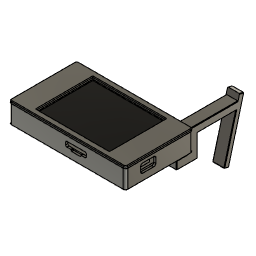
Cheap Yellow Display v16 (Autodesk Fusion 360 design; units mm, degrees)
part number: CYD
Autodesk Fusion 360 part; units mm, degrees
(part 1 of 2)
sketch "Sketch1" plane through (0, 0, 0) normal (0, 0, 1) x (1, 0, 0) in component "Display"
  line L0 (-39, 21) -> (39, 21) construction
  line L1 (39, 21) -> (39, -21) construction
  line L2 (39, -21) -> (-39, -21) construction
  line L3 (-39, -21) -> (-39, 21) construction
  line L4 (39, -25) -> (-39, -25)
  line L5 (-43, -21) -> (-43, 21)
  line L6 (-39, 25) -> (39, 25)
  line L7 (43, 21) -> (43, -21)
  arc A0 (43, 21) -> (39, 25) centre (39, 21) ccw
  arc A1 (39, -25) -> (43, -21) centre (39, -21) ccw
  arc A2 (-43, -21) -> (-39, -25) centre (-39, -21) ccw
  arc A3 (-39, 25) -> (-43, 21) centre (-39, 21) ccw
  circle A4 centre (-39, -21) radius 1.6
  circle A5 centre (39, -21) radius 1.6
  circle A6 centre (39, 21) radius 1.6
  circle A7 centre (-39, 21) radius 1.6
  dimension "d1" = 78
  dimension "d2" = 42
  dimension "d4" = 4
  dimension "d5" = 4
  dimension "d6" = 4
  dimension "d7" = 4
  dimension "d8" = 3.2
  dimension "d9" = 3.2
  dimension "d10" = 3.2
  dimension "d11" = 3.2
  constraint horizontal L0
  constraint vertical L1
  constraint horizontal L2
  constraint vertical L3
  constraint tangent L6 A0
  constraint tangent L7 A0
  constraint tangent L7 A1
  constraint tangent L4 A1
  constraint tangent L4 A2
  constraint tangent L5 A2
  constraint tangent L5 A3
  constraint tangent L6 A3
  constraint concentric A2 A4
  constraint concentric A1 A5
  constraint concentric A0 A6
  constraint concentric A3 A7
  measures "d1" distance of L0.start L0.end
  measures "d2" distance of L0.start L2.end
  measures "d4" radius of A0
  measures "d5" radius of A1
  measures "d6" radius of A2
  measures "d7" radius of A3
  measures "d8" diameter of A4
  measures "d9" diameter of A5
  measures "d10" diameter of A6
  measures "d11" diameter of A7
extrude "Extrude1" add sketch "Sketch1" along normal blind 1.5 makes body 1 in component "Display"
sketch "Sketch2" plane through (0, 0, 1.5) normal (0, 0, 1) x (-1, 0, 0) in component "Display"
  circle A0 centre (-39, 21) radius 1.6
  circle A1 centre (39, -21) radius 1.6
  circle A2 centre (39, 21) radius 1.6
  circle A3 centre (-39, -21) radius 1.6
  arc A4 (-43, -21) -> (-39, -25) centre (-39, -21) ccw
  line L0 (-39, -25) -> (39, -25)
  arc A5 (39, -25) -> (43, -21) centre (39, -21) ccw
  line L1 (43, -21) -> (43, 21)
  arc A6 (43, 21) -> (39, 25) centre (39, 21) ccw
  line L2 (39, 25) -> (-39, 25)
  arc A7 (-39, 25) -> (-43, 21) centre (-39, 21) ccw
  line L3 (-43, 21) -> (-43, -21)
  line L4 (34.5, -25) -> (-34.5, -25)
  line L5 (-34.5, -25) -> (-34.5, 25)
  line L6 (-34.5, 25) -> (34.5, 25)
  line L7 (34.5, 25) -> (34.5, -25)
  line L8 (41, 11) -> (38, 11)
  line L9 (38, 11) -> (38, 17)
  line L10 (38, 17) -> (41, 17)
  line L11 (41, 17) -> (41, 11)
  dimension "d14" = 69
  dimension "d15" = 50
  dimension "d16" = 8.5
  dimension "d19" = 6
  dimension "d20" = 2
  dimension "d21" = 8
  constraint horizontal L4
  constraint vertical L5
  constraint horizontal L6
  constraint vertical L7
  constraint horizontal L8
  constraint vertical L9
  constraint horizontal L10
  constraint vertical L11
  measures "d14" distance of L4.start L4.end
  measures "d15" distance of L4.start L6.end
  measures "d16" distance of L3 L5
  measures "d19" distance of L8.start L10.end
  measures "d20" distance of L1 L11
  measures "d21" distance of L2 L10
extrude "Extrude2" add sketch "Sketch2" along normal blind 3.5 contours L0 L2 L4 L5 L6 L7 bodies 1 in component "Display"
extrude "Extrude3" add sketch "Sketch2" along normal blind 0.5 contours L8 L9 L10 L11 bodies 1 in component "Display"
sketch "Sketch3" plane through (0, 0, 0) normal (0, 0, -1) x (1, 0, 0) in component "Display"
  circle A0 centre (39, 21) radius 1.6
  circle A1 centre (-39, -21) radius 1.6
  circle A2 centre (-39, 21) radius 1.6
  circle A3 centre (39, -21) radius 1.6
  arc A4 (39, -25) -> (43, -21) centre (39, -21) ccw
  line L0 (43, -21) -> (43, 21)
  arc A5 (43, 21) -> (39, 25) centre (39, 21) ccw
  line L1 (39, 25) -> (-39, 25)
  arc A6 (-39, 25) -> (-43, 21) centre (-39, 21) ccw
  line L2 (-43, 21) -> (-43, -21)
  arc A7 (-43, -21) -> (-39, -25) centre (-39, -21) ccw
  line L3 (-39, -25) -> (39, -25)
  line L4 (-17.6, -9) -> (-43, -9)
  line L5 (-43, -9) -> (-43, 9)
  line L6 (-43, 9) -> (-17.6, 9)
  line L7 (-17.6, 9) -> (-17.6, -9)
  line L8 (-10, 11.5) -> (-15, 11.5)
  line L9 (-15, 11.5) -> (-15, 16.5)
  line L10 (-15, 16.5) -> (-10, 16.5)
  line L11 (-10, 16.5) -> (-10, 11.5)
  line L12 (-31.9, -23.2) -> (-35.4, -23.2)
  line L13 (-35.4, -23.2) -> (-35.4, -17.2)
  line L14 (-35.4, -17.2) -> (-31.9, -17.2)
  line L15 (-31.9, -17.2) -> (-31.9, -23.2)
  line L16 (-31.4, -23.2) -> (-31.4, -17.2)
  line L17 (-31.4, -17.2) -> (-27.9, -17.2)
  line L18 (-27.9, -17.2) -> (-27.9, -23.2)
  line L19 (-27.9, -23.2) -> (-31.4, -23.2)
  line L20 (19, -23.8) -> (11.4, -23.8)
  line L21 (11.4, -23.8) -> (11.4, -20.6)
  line L22 (11.4, -20.6) -> (19, -20.6)
  line L23 (19, -20.6) -> (19, -23.8)
  line L24 (-36, -9) -> (-36, 9)
  line L25 (42, -14) -> (37.5, -14)
  line L26 (37.5, -14) -> (37.5, -4)
  line L27 (37.5, -4) -> (42, -4)
  line L28 (42, -4) -> (42, -14)
  line L29 (43.6, 5.4) -> (38.1, 5.4)
  line L30 (38.1, 5.4) -> (38.1, 13.2)
  line L31 (38.1, 13.2) -> (43.6, 13.2)
  line L32 (43.6, 13.2) -> (43.6, 5.4)
  line L33 (-22.8, 20.6) -> (-32.8, 20.6)
  line L34 (-32.8, 20.6) -> (-32.8, 24.9)
  line L35 (-32.8, 24.9) -> (-22.8, 24.9)
  line L36 (-22.8, 24.9) -> (-22.8, 20.6)
  line L37 (-16.8, 20.6) -> (-16.8, 24.9)
  line L38 (-16.8, 24.9) -> (-6.8, 24.9)
  line L39 (-6.8, 24.9) -> (-6.8, 20.6)
  line L40 (-6.8, 20.6) -> (-16.8, 20.6)
  line L41 (-2.6, 24.9) -> (12.4, 24.9)
  line L42 (12.4, 24.9) -> (12.4, 9.9)
  line L43 (12.4, 9.9) -> (-2.6, 9.9)
  line L44 (-2.6, 9.9) -> (-2.6, 24.9)
  dimension "d24" = 25.4
  dimension "d25" = 18
  dimension "d26" = 16
  dimension "d27" = 5
  dimension "d28" = 8.5
  dimension "d29" = 28
  dimension "d33" = 3.5
  dimension "d34" = 6
  dimension "d35" = 7.6
  dimension "d36" = 1.8
  dimension "d37" = 3.5
  dimension "d38" = 6
  dimension "d39" = 7.6
  dimension "d40" = 3.2
  dimension "d41" = 1.2
  dimension "d42" = 24
  dimension "d43" = 7
  dimension "d44" = 4.5
  dimension "d45" = 10
  dimension "d46" = 1
  dimension "d47" = 11
  dimension "d48" = 5.5
  dimension "d49" = 7.8
  dimension "d50" = 0.6
  dimension "d51" = 11.8
  dimension "d52" = 10
  dimension "d53" = 4.3
  dimension "d54" = 10.2
  dimension "d55" = 10
  dimension "d56" = 4.3
  dimension "d92" = 0.1
  dimension "d93" = 40.4
  constraint horizontal L4
  constraint vertical L5
  constraint horizontal L6
  constraint vertical L7
  constraint horizontal L8
  constraint vertical L9
  constraint horizontal L10
  constraint vertical L11
  constraint horizontal L12
  constraint vertical L13
  constraint horizontal L14
  constraint vertical L15
  constraint horizontal L19
  constraint vertical L16
  constraint horizontal L17
  constraint vertical L18
  constraint horizontal L20
  constraint vertical L21
  constraint horizontal L22
  constraint vertical L23
  constraint coincident L4 L24.start
  constraint coincident L6 L24.end
  constraint perpendicular L6 L24
  constraint horizontal L25
  constraint vertical L26
  constraint horizontal L27
  constraint vertical L28
  constraint horizontal L29
  constraint vertical L30
  constraint horizontal L31
  constraint vertical L32
  constraint horizontal L33
  constraint vertical L34
  constraint horizontal L35
  constraint vertical L36
  constraint horizontal L40
  constraint vertical L37
  constraint horizontal L38
  constraint vertical L39
  constraint horizontal L41
  constraint vertical L42
  constraint horizontal L43
  constraint vertical L44
  measures "d24" distance of L4.start L4.end
  measures "d25" distance of L4.start L6.end
  measures "d26" distance of L1 L6
  measures "d27" distance of L8.start L8.end
  measures "d28" distance of L1 L9.end
  measures "d29" distance of L2 L9.end
  measures "d33" distance of L12.start L12.end
  measures "d34" distance of L12.start L14.end
  measures "d35" horizontal distance of L2.end L12.end
  measures "d36" vertical distance of A7.end L12.end
  measures "d37" distance of L16.start L18.end
  measures "d38" distance of L18.end L17.end
  measures "d39" distance of L20.start L20.end
  measures "d40" distance of L20.start L22.end
  measures "d41" distance of L3 L20.end
  measures "d42" distance of A4.end L23
  measures "d43" distance of L5 L24
  measures "d44" distance of L25.start L25.end
  measures "d45" distance of L25.start L27.end
  measures "d46" distance of L0 L28
  measures "d47" distance of L3 L25
  measures "d48" distance of L29.start L29.end
  measures "d49" distance of L29.start L31.end
  measures "d50" distance of L0 L32
  measures "d51" distance of L1 L31
  measures "d52" distance of L33.start L33.end
  measures "d53" distance of L33.start L35.end
  measures "d54" distance of A6.end L34
  measures "d55" distance of L39.end L37.start
  measures "d56" distance of L38.end L39.end
  measures "d92" distance of L1 L41
  measures "d93" distance of L2 L44
extrude "Extrude4" add sketch "Sketch3" along normal blind 3 contours L4 L6 L7 L24 bodies 1 in component "Display"
extrude "Extrude5" add sketch "Sketch3" along normal blind 1 contours L2 L4 L5 L6 L24 bodies 1 in component "Display"
extrude "Extrude6" add sketch "Sketch3" along normal blind 3.5 contours L25 L26 L27 L28 | L33 L34 L35 L36 | L37 L38 L39 L40 bodies 1 in component "Display"
extrude "Extrude7" add sketch "Sketch3" along normal blind 1.5 contours L8 L9 L10 L11 bodies 1 in component "Display"
extrude "Extrude8" add sketch "Sketch3" along normal blind 2.5 contours L0 L29 L30 L31 | L0 L29 L31 L32 bodies 1 in component "Display"
extrude "Extrude9" add sketch "Sketch3" along normal blind 1.8 contours L41 L42 L43 L44 bodies 1 in component "Display"
extrude "Extrude10" add sketch "Sketch3" along normal blind 4.6 contours L20 L21 L22 L23 bodies 1 in component "Display"
extrude "Extrude11" add sketch "Sketch3" along normal blind 3.7 contours L12 L13 L14 L15 | L16 L17 L18 L19 bodies 1 in component "Display"
sketch "Sketch4" plane through (0, 0, -3.7) normal (0, 0, -1) x (1, 0, 0) in component "Display"
  line L0 (-27.9, -23.2) -> (-27.9, -17.2)
  line L1 (-27.9, -17.2) -> (-31.4, -17.2)
  line L2 (-31.4, -17.2) -> (-31.4, -23.2)
  line L3 (-31.4, -23.2) -> (-27.9, -23.2)
  line L4 (-28.9, -21.7) -> (-30.4, -21.7)
  line L5 (-30.4, -21.7) -> (-30.4, -18.7)
  line L6 (-30.4, -18.7) -> (-28.9, -18.7)
  line L7 (-28.9, -18.7) -> (-28.9, -21.7)
  line L8 (-29.65, -23.2) -> (-29.65, -24) construction
  line L9 (-31.4, -20.2) -> (-32, -20.2) construction
  line L10 (-35.4, -17.2) -> (-31.9, -17.2)
  line L11 (-31.9, -17.2) -> (-31.9, -23.2)
  line L12 (-35.4, -23.2) -> (-35.4, -17.2)
  line L13 (-31.9, -23.2) -> (-35.4, -23.2)
  line L14 (-33.65, -23.2) -> (-33.65, -24) construction
  line L15 (-35.4, -20.2) -> (-36, -20.2) construction
  line L16 (-34.4, -18.7) -> (-32.9, -18.7)
  line L17 (-32.9, -18.7) -> (-32.9, -21.7)
  line L18 (-32.9, -21.7) -> (-34.4, -21.7)
  line L19 (-34.4, -21.7) -> (-34.4, -18.7)
  dimension "d73" = 1.5
  dimension "d74" = 3
  dimension "d75" = 1.5
  dimension "d76" = 3
  constraint horizontal L4
  constraint vertical L5
  constraint horizontal L6
  constraint vertical L7
  constraint midpoint L3 L8.start
  constraint perpendicular L3 L8
  constraint midpoint L2 L9.start
  constraint perpendicular L2 L9
  constraint symmetric L5 L7 L8
  constraint symmetric L4 L6 L9
  constraint midpoint L13 L14.start
  constraint perpendicular L13 L14
  constraint midpoint L12 L15.start
  constraint perpendicular L12 L15
  constraint horizontal L18
  constraint vertical L19
  constraint horizontal L16
  constraint vertical L17
  constraint symmetric L15 L16 L18
  constraint symmetric L14 L17 L19
  measures "d73" distance of L4.start L4.end
  measures "d74" distance of L4.start L6.end
  measures "d75" distance of L17.end L18.end
  measures "d76" distance of L17.end L16.end
extrude "Extrude12" add sketch "Sketch4" along normal blind 1 contours L4 L5 L6 L7 | L16 L17 L18 L19 bodies 1 in component "Display"
sketch "Sketch5" plane through (0, 0, -1.5) normal (0, 0, -1) x (1, 0, 0) in component "Display"
  line L0 (-10, 16.5) -> (-15, 16.5)
  line L1 (-15, 16.5) -> (-15, 11.5)
  line L2 (-15, 11.5) -> (-10, 11.5)
  line L3 (-10, 11.5) -> (-10, 16.5)
  line L4 (-15, 16.5) -> (-10, 16.5)
  line L5 (-10, 16.5) -> (-10, 11.5)
  line L6 (-15, 11.5) -> (-15, 16.5)
  line L7 (-10, 11.5) -> (-15, 11.5)
  line L8 (-15, 16.5) -> (-10, 11.5) construction
  circle A0 centre (-12.5, 14) radius 2
  dimension "d79" = 4
  constraint coincident L0.end L1.start
  constraint coincident L2.end L3.start
  constraint midpoint L8 A0.centre
  measures "d79" diameter of A0
extrude "Extrude13" add sketch "Sketch5" along normal blind 0.1 contours A0 bodies 1 in component "Display"
sketch "Sketch6" plane through (0, 0, 5) normal (0, 0, 1) x (-1, 0, 0) in component "Display"
  line L0 (34.5, 25) -> (-34.5, 25)
  line L1 (-34.5, 25) -> (-34.5, -25)
  line L2 (-34.5, -25) -> (34.5, -25)
  line L3 (34.5, -25) -> (34.5, 25)
  line L4 (32, -22.5) -> (-27, -22.5)
  line L5 (-27, -22.5) -> (-27, 22.5)
  line L6 (-27, 22.5) -> (32, 22.5)
  line L7 (32, 22.5) -> (32, -22.5)
  line L8 (34.5, 0) -> (42, 0) construction
  line L9 (43, -21) -> (43, 21)
  line L10 (43, -9.5) -> (36.8, -9.5)
  line L11 (36.8, -9.5) -> (36.8, 9.5)
  line L12 (36.8, 9.5) -> (43, 9.5)
  line L13 (43, 9.5) -> (43, -9.5)
  dimension "d82" = 59
  dimension "d83" = 45
  dimension "d84" = 2.5
  dimension "d85" = 6.2
  dimension "d86" = 19
  constraint horizontal L4
  constraint vertical L5
  constraint horizontal L6
  constraint vertical L7
  constraint midpoint L3 L8.start
  constraint perpendicular L3 L8
  constraint symmetric L4 L6 L8
  constraint horizontal L10
  constraint vertical L11
  constraint horizontal L12
  constraint vertical L13
  constraint coincident L9 L10.start
  constraint symmetric L8 L10 L12
  measures "d82" distance of L4.start L4.end
  measures "d83" distance of L4.start L6.end
  measures "d84" distance of L3 L7
  measures "d85" distance of L10.start L10.end
  measures "d86" distance of L10.start L12.end
extrude "Extrude14" add sketch "Sketch6" along normal blind 0.1 contours L4 L5 L6 L7 bodies 1 in component "Display"
extrude "Extrude15" cut sketch "Sketch6" against normal up to surface (1.5 mm away) from surface at -3.5 contours L9 L10 L11 L12 L13 bodies 1 in component "Display"
sketch "Sketch1 (2)" plane through (0, 0, 5) normal (0, 0, 1) x (-1, 0, 0) in component "case front"
  line L0 (32, 22.5) -> (32, -22.5)
  line L1 (32, -22.5) -> (-27, -22.5)
  line L2 (-27, -22.5) -> (-27, 22.5)
  line L3 (-27, 22.5) -> (32, 22.5)
  line L4 (34.5, 25) -> (-34.5, 25)
  line L5 (-34.5, 25) -> (-34.5, -25)
  line L6 (-34.5, -25) -> (34.5, -25)
  line L7 (34.5, -25) -> (34.5, 25)
  line L8 (-27, 22.5) -> (-27, -22.5)
  line L9 (-27, -22.5) -> (32, -22.5)
  line L10 (32, -22.5) -> (32, 22.5)
  line L11 (32, 22.5) -> (-27, 22.5)
  line L12 (-27, 22.5) -> (-27, -22.5)
  line L13 (-27, -22.5) -> (32, -22.5)
  line L14 (32, -22.5) -> (32, 22.5)
  line L15 (-28, 23.5) -> (33, 23.5)
  line L16 (33, 23.5) -> (33, -23.5)
  line L17 (33, -23.5) -> (-28, -23.5)
  line L18 (-28, -23.5) -> (-28, 23.5)
  line L19 (43, -21) -> (43, -9.5) construction
  line L20 (-34.5, -25) -> (34.5, -25)
  line L21 (34.5, 25) -> (-34.5, 25)
  line L22 (-43, 21) -> (-43, -21) construction
  line L23 (49.5, -28.5) -> (-44.5, -28.5)
  line L24 (-46.5, -26.5) -> (-46.5, 26.5)
  line L25 (-44.5, 28.5) -> (49.5, 28.5)
  line L26 (51.5, 26.5) -> (51.5, -26.5)
  arc A0 (51.5, 26.5) -> (49.5, 28.5) centre (49.5, 26.5) ccw
  arc A1 (49.5, -28.5) -> (51.5, -26.5) centre (49.5, -26.5) ccw
  arc A2 (-46.5, -26.5) -> (-44.5, -28.5) centre (-44.5, -26.5) ccw
  arc A3 (-44.5, 28.5) -> (-46.5, 26.5) centre (-44.5, 26.5) ccw
  dimension "d94" = -1
  dimension "d99" = 2
  dimension "d100" = 2
  dimension "d101" = 2
  dimension "d102" = 2
  dimension "d105" = 18.5
  dimension "d106" = 18.5
  dimension "BORDER_H" = 5
  dimension "d108" = 5
  constraint horizontal L23
  constraint vertical L24
  constraint horizontal L25
  constraint vertical L26
  constraint tangent L26 A0
  constraint tangent L25 A0
  constraint tangent L26 A1
  constraint tangent L23 A1
  constraint tangent L23 A2
  constraint tangent L24 A2
  constraint tangent L24 A3
  constraint tangent L25 A3
  measures "d99" radius of A0
  measures "d100" radius of A1
  measures "d101" radius of A2
  measures "d102" radius of A3
  measures "d105" distance of L16 L26
  measures "d106" distance of L18 L24
  measures "BORDER_H" distance of L17 L23
  measures "d108" distance of L15 L25
extrude "Extrude1'" add sketch "Sketch1 (2)" along normal blind 1.8 separate body contours L4 L5 L6 L7 L20 L21 | L23 L24 L25 L26 A0 A1 A2 A3 makes body 2 in component "case front"
sketch "Sketch2 (2)" plane through (0, 0, 5) normal (0, 0, -1) x (1, 0, 0) in component "case front"
  line L0 (28, -23.5) -> (-33, -23.5)
  line L1 (-33, -23.5) -> (-33, 23.5)
  line L2 (-33, 23.5) -> (28, 23.5)
  line L3 (28, 23.5) -> (28, -23.5)
  arc A0 (-49.5, 28.5) -> (-51.5, 26.5) centre (-49.5, 26.5) ccw
  line L4 (-51.5, 26.5) -> (-51.5, -26.5)
  arc A1 (-51.5, -26.5) -> (-49.5, -28.5) centre (-49.5, -26.5) ccw
  line L5 (-49.5, -28.5) -> (44.5, -28.5)
  arc A2 (44.5, -28.5) -> (46.5, -26.5) centre (44.5, -26.5) ccw
  line L6 (46.5, -26.5) -> (46.5, 26.5)
  arc A3 (46.5, 26.5) -> (44.5, 28.5) centre (44.5, 26.5) ccw
  line L7 (44.5, 28.5) -> (-49.5, 28.5)
  line L8 (44.5, 28.5) -> (-49.5, 28.5)
  arc A4 (46.5, 26.5) -> (44.5, 28.5) centre (44.5, 26.5) ccw
  line L9 (46.5, -26.5) -> (46.5, 26.5)
  arc A5 (44.5, -28.5) -> (46.5, -26.5) centre (44.5, -26.5) ccw
  line L10 (-49.5, -28.5) -> (44.5, -28.5)
  arc A6 (-51.5, -26.5) -> (-49.5, -28.5) centre (-49.5, -26.5) ccw
  line L11 (-51.5, 26.5) -> (-51.5, -26.5)
  arc A7 (-49.5, 28.5) -> (-51.5, 26.5) centre (-49.5, 26.5) ccw
  line L12 (-50.5, 26.5) -> (-50.5, -26.5)
  arc A8 (-50.5, -26.5) -> (-49.5, -27.5) centre (-49.5, -26.5) ccw
  line L13 (-49.5, -27.5) -> (44.5, -27.5)
  arc A9 (44.5, -27.5) -> (45.5, -26.5) centre (44.5, -26.5) ccw
  line L14 (45.5, -26.5) -> (45.5, 26.5)
  arc A10 (45.5, 26.5) -> (44.5, 27.5) centre (44.5, 26.5) ccw
  line L15 (44.5, 27.5) -> (-49.5, 27.5)
  arc A11 (-49.5, 27.5) -> (-50.5, 26.5) centre (-49.5, 26.5) ccw
  line L16 (-49.7, 26.5) -> (-49.7, -26.5)
  arc A12 (-49.7, -26.5) -> (-49.5, -26.7) centre (-49.5, -26.5) ccw
  line L17 (-49.5, -26.7) -> (44.5, -26.7)
  arc A13 (44.5, -26.7) -> (44.7, -26.5) centre (44.5, -26.5) ccw
  line L18 (44.7, -26.5) -> (44.7, 26.5)
  arc A14 (44.7, 26.5) -> (44.5, 26.7) centre (44.5, 26.5) ccw
  line L19 (44.5, 26.7) -> (-49.5, 26.7)
  arc A15 (-49.5, 26.7) -> (-49.7, 26.5) centre (-49.5, 26.5) ccw
  circle A16 centre (-39, -21) radius 1.6
  circle A17 centre (-39, 21) radius 1.6
  circle A18 centre (39, 21) radius 1.6
  circle A19 centre (39, -21) radius 1.6
  circle A20 centre (39, 21) radius 3.6
  circle A21 centre (-39, 21) radius 3.6
  circle A22 centre (-39, -21) radius 3.6
  circle A23 centre (39, -21) radius 3.6
  circle A24 centre (-39, 21) radius 1.4
  circle A25 centre (39, 21) radius 1.4
  circle A26 centre (39, -21) radius 1.4
  circle A27 centre (-39, -21) radius 1.4
  dimension "d110" = -1
  dimension "d112" = 2
  dimension "d113" = 2
  dimension "d114" = 2
  dimension "d115" = 2
  dimension "d116" = -0.2
  dimension "d117" = -0.2
  dimension "d118" = -0.2
  dimension "d119" = -0.2
extrude "Extrude2'" add sketch "Sketch2 (2)" along normal blind 1 contours L12 A8 L13 A9 L14 A10 L15 A11 bodies 2 in component "case front"
extrude "Extrude3'" add sketch "Sketch2 (2)" along normal up to surface (5 mm away) contours A16 | A17 | A18 | A19 | A24 | A25 | A26 | A27 bodies 2 in component "case front"
extrude "Extrude4'" add sketch "Sketch2 (2)" along normal up to surface (3.5 mm away) contours A20 | A21 | A22 | A23 bodies 2 in component "case front"
chamfer "Chamfer1" distance 0.6 angle 45 12 edges at (45.9142, 27.9142, 6.8) (-2.5, 28.5, 6.8) (-50.9142, 27.9142, 6.8) (-51.5, 0, 6.8) (-50.9142, -27.9142, 6.8) (-2.5, -28.5, 6.8) (45.9142, -27.9142, 6.8) (46.5, 0, 6.8) (-33, 0, 6.8) (-2.5, -23.5, 6.8) (-2.5, 23.5, 6.8) (28, 0, 6.8) on bodies 2 in component "case front"
sketch "Sketch1 (3)" plane through (0, 0, 4) normal (0, 0, -1) x (1, 0, 0) in component "case rear"
  arc A0 (-49.5, 26.7) -> (-49.7, 26.5) centre (-49.5, 26.5) ccw
  line L0 (-49.5, 26.7) -> (44.5, 26.7)
  arc A1 (44.7, 26.5) -> (44.5, 26.7) centre (44.5, 26.5) ccw
  line L1 (44.7, 26.5) -> (44.7, -26.5)
  arc A2 (44.5, -26.7) -> (44.7, -26.5) centre (44.5, -26.5) ccw
  line L2 (44.5, -26.7) -> (-49.5, -26.7)
  arc A3 (-49.7, -26.5) -> (-49.5, -26.7) centre (-49.5, -26.5) ccw
  line L3 (-49.7, -26.5) -> (-49.7, 26.5)
  arc A4 (-49.5, 27.5) -> (-50.5, 26.5) centre (-49.5, 26.5) ccw
  line L4 (-50.5, 26.5) -> (-50.5, -26.5)
  arc A5 (-50.5, -26.5) -> (-49.5, -27.5) centre (-49.5, -26.5) ccw
  line L5 (-49.5, -27.5) -> (44.5, -27.5)
  arc A6 (44.5, -27.5) -> (45.5, -26.5) centre (44.5, -26.5) ccw
  line L6 (45.5, -26.5) -> (45.5, 26.5)
  arc A7 (45.5, 26.5) -> (44.5, 27.5) centre (44.5, 26.5) ccw
  line L7 (44.5, 27.5) -> (-49.5, 27.5)
  arc A8 (-51.5, -26.5) -> (-49.5, -28.5) centre (-49.5, -26.5) ccw
  line L8 (-49.5, -28.5) -> (44.5, -28.5)
  line L9 (-51.5, 26.5) -> (-51.5, -26.5)
  arc A9 (44.5, -28.5) -> (46.5, -26.5) centre (44.5, -26.5) ccw
  line L10 (46.5, -26.5) -> (46.5, 26.5)
  arc A10 (46.5, 26.5) -> (44.5, 28.5) centre (44.5, 26.5) ccw
  line L11 (44.5, 28.5) -> (-49.5, 28.5)
  arc A11 (-49.5, 28.5) -> (-51.5, 26.5) centre (-49.5, 26.5) ccw
  line L12 (-49.7, -26.5) -> (-49.7, 26.5)
  arc A12 (-49.5, 26.7) -> (-49.7, 26.5) centre (-49.5, 26.5) ccw
  line L13 (-49.5, 26.7) -> (44.5, 26.7)
  arc A13 (44.7, 26.5) -> (44.5, 26.7) centre (44.5, 26.5) ccw
  line L14 (44.7, 26.5) -> (44.7, -26.5)
  arc A14 (44.5, -26.7) -> (44.7, -26.5) centre (44.5, -26.5) ccw
  line L15 (44.5, -26.7) -> (-49.5, -26.7)
  arc A15 (-49.7, -26.5) -> (-49.5, -26.7) centre (-49.5, -26.5) ccw
  arc A16 (44.5, -27.7) -> (45.7, -26.5) centre (44.5, -26.5) ccw
  line L16 (45.7, -26.5) -> (45.7, 26.5)
  arc A17 (45.7, 26.5) -> (44.5, 27.7) centre (44.5, 26.5) ccw
  line L17 (44.5, 27.7) -> (-49.5, 27.7)
  arc A18 (-49.5, 27.7) -> (-50.7, 26.5) centre (-49.5, 26.5) ccw
  line L18 (-50.7, 26.5) -> (-50.7, -26.5)
  arc A19 (-50.7, -26.5) -> (-49.5, -27.7) centre (-49.5, -26.5) ccw
  line L19 (-49.5, -27.7) -> (44.5, -27.7)
  dimension "d127" = -0.8
extrude "Extrude1''" add sketch "Sketch1 (3)" against normal up to surface (0.9 mm away) separate body contours A8 L8 L9 A9 L10 A10 L11 A11 makes body 3 in component "case rear"
extrude "Extrude2''" add sketch "Sketch1 (3)" along normal blind 15 contours A4 L4 A5 L5 A6 L6 A7 L7 | A8 L8 L9 A9 L10 A10 L11 A11 | A16 L16 A17 L17 A18 L18 A19 L19 bodies 3 in component "case rear"
sketch "Sketch2 (3)" plane through (0, 0, -11) normal (0, 0, -1) x (1, 0, 0) in component "case rear"
  arc A0 (-49.5, 26.7) -> (-49.7, 26.5) centre (-49.5, 26.5) ccw
  line L0 (-49.5, 26.7) -> (44.5, 26.7)
  arc A1 (44.7, 26.5) -> (44.5, 26.7) centre (44.5, 26.5) ccw
  line L1 (44.7, 26.5) -> (44.7, -26.5)
  arc A2 (44.5, -26.7) -> (44.7, -26.5) centre (44.5, -26.5) ccw
  line L2 (44.5, -26.7) -> (-49.5, -26.7)
  arc A3 (-49.7, -26.5) -> (-49.5, -26.7) centre (-49.5, -26.5) ccw
  line L3 (-49.7, -26.5) -> (-49.7, 26.5)
  arc A4 (-49.5, 28.5) -> (-51.5, 26.5) centre (-49.5, 26.5) ccw
  line L4 (-51.5, 26.5) -> (-51.5, -26.5)
  arc A5 (-51.5, -26.5) -> (-49.5, -28.5) centre (-49.5, -26.5) ccw
  line L5 (-49.5, -28.5) -> (44.5, -28.5)
  arc A6 (44.5, -28.5) -> (46.5, -26.5) centre (44.5, -26.5) ccw
  line L6 (46.5, -26.5) -> (46.5, 26.5)
  arc A7 (46.5, 26.5) -> (44.5, 28.5) centre (44.5, 26.5) ccw
  line L7 (44.5, 28.5) -> (-49.5, 28.5)
  line L8 (46.5, -26.5) -> (46.5, 26.5)
  arc A8 (46.5, 26.5) -> (44.5, 28.5) centre (44.5, 26.5) ccw
  line L9 (44.5, 28.5) -> (-49.5, 28.5)
  arc A9 (-49.5, 28.5) -> (-51.5, 26.5) centre (-49.5, 26.5) ccw
  line L10 (-51.5, 26.5) -> (-51.5, -26.5)
  arc A10 (-51.5, -26.5) -> (-49.5, -28.5) centre (-49.5, -26.5) ccw
  arc A11 (44.5, -28.5) -> (46.5, -26.5) centre (44.5, -26.5) ccw
  line L11 (-49.5, -28.5) -> (44.5, -28.5)
  circle A12 centre (-39, -21) radius 1.6
  circle A13 centre (39, -21) radius 1.6
  circle A14 centre (39, 21) radius 1.6
  circle A15 centre (-39, 21) radius 1.6
  circle A16 centre (-44, -21) radius 3.4
  circle A17 centre (-44, 21) radius 3.4
  circle A18 centre (39, -21) radius 3.4
  circle A19 centre (39, 21) radius 3.4
  line L12 (-44, -21) -> (39, -21)
  line L13 (39, -21) -> (39, 21)
  line L14 (39, 21) -> (-44, 21)
  line L15 (-44, 21) -> (-44, -21)
  circle A20 centre (-44, -21) radius 5
  circle A21 centre (-44, 21) radius 5
  circle A22 centre (39, -21) radius 5
  circle A23 centre (39, 21) radius 5
  point P0 (39, -21)
  dimension "d132" = 1.8
  dimension "d133" = 1.8
  dimension "d134" = 1.8
  dimension "d135" = 1.8
  dimension "d210" = 10
  dimension "d211" = 10
  dimension "d212" = 10
  dimension "d213" = 10
  constraint horizontal L12
  constraint vertical L13
  constraint horizontal L14
  constraint vertical L15
  constraint coincident A14.centre A19.centre
  constraint coincident A16.centre L12.start
  constraint concentric A16 A20
  constraint concentric A17 A21
  constraint concentric A13 A22
  constraint coincident P0 A13.centre
  measures "d210" diameter of A20
  measures "d211" diameter of A21
  measures "d212" diameter of A22
  measures "d213" diameter of A23
extrude "Extrude3''" add sketch "Sketch2 (3)" against normal up to surface (10.9 mm away) separate body contours A16 L12 L15 | A16 L12 L15 | A13 A18 L12 L13 | A13 A18 L12 L13 | A13 L12 L13 | A13 L12 L13 | A17 L14 L15 | A17 L14 L15 | A14 A19 L13 L14 | A14 A19 L13 L14 | A14 L13 L14 | A14 L13 L14 makes body 4 at (-40.6169, 20.6615, -7.3667) makes body 5 at (42.3831, 20.6615, -7.3667) makes body 6 at (-40.6169, -21.3385, -7.3667) makes body 7 at (42.3831, -21.3385, -7.3667) in component "case rear"
extrude "Extrude4''" add sketch "Sketch2 (3)" against normal blind 1.8 contours A0 L0 A1 L1 A2 L2 A3 L3 | A12 L12 A20 | A12 L12 A20 | A12 A15 L12 L13 L14 L15 A20 A21 A22 A23 | A12 L12 A20 | A12 A16 L15 A20 | A12 A16 L15 A20 | A12 L12 A20 | A18 L12 L13 A22 | A18 L12 L13 A22 | A15 A17 L15 A21 | A15 A17 L15 A21 | A19 L13 L14 A23 | A19 L13 L14 A23 | A15 L14 A21 | A15 L14 A21 | A15 L14 A21 | A15 L14 A21 bodies 3 4 5 6 7 in component "case rear"
sketch "Sketch3 (2)" plane through (46.5, 0, 0) normal (1, 0, 0) x (0, 1, 0) in component "case rear"
  line L0 (26.5, 4.9) -> (-26.5, 4.9)
  line L1 (-26.5, 4.9) -> (-26.5, -11)
  line L2 (-26.5, -11) -> (26.5, -11)
  line L3 (26.5, -11) -> (26.5, 4.9)
  line L4 (-5.4, 0) -> (-13.2, 0)
  line L5 (-13.2, 0) -> (-13.2, -2.5)
  line L6 (-13.2, -2.5) -> (-5.4, -2.5)
  line L7 (-5.4, -2.5) -> (-5.4, 0)
  line L8 (-14.1, -5) -> (-4.5, -5)
  line L9 (-2.9, -3.4) -> (-2.9, 0.9)
  line L10 (-4.5, 2.5) -> (-14.1, 2.5)
  line L11 (-15.7, 0.9) -> (-15.7, -3.4)
  arc A0 (-14.1, 2.5) -> (-15.7, 0.9) centre (-14.1, 0.9) ccw
  arc A1 (-2.9, 0.9) -> (-4.5, 2.5) centre (-4.5, 0.9) ccw
  arc A2 (-4.5, -5) -> (-2.9, -3.4) centre (-4.5, -3.4) ccw
  arc A3 (-15.7, -3.4) -> (-14.1, -5) centre (-14.1, -3.4) ccw
  dimension "d141" = 1.6
  dimension "d142" = 1.6
  dimension "d143" = 1.6
  dimension "d144" = 1.6
  constraint tangent L11 A0
  constraint tangent L10 A0
  constraint tangent L10 A1
  constraint tangent L9 A1
  constraint tangent L9 A2
  constraint tangent L8 A2
  constraint tangent L8 A3
  constraint tangent L11 A3
  measures "d141" radius of A0
  measures "d142" radius of A1
  measures "d143" radius of A2
  measures "d144" radius of A3
extrude "Extrude5'" cut sketch "Sketch3 (2)" against normal up to surface (1.8 mm away) contours L4 L5 L6 L7 | L8 L9 L10 L11 A0 A1 A2 A3 bodies 3 in component "case rear"
chamfer "Chamfer1'" distance 0.6 angle 45 8 edges at (-2.5, 28.5, -11) (45.9142, 27.9142, -11) (46.5, 0, -11) (45.9142, -27.9142, -11) (-2.5, -28.5, -11) (-50.9142, -27.9142, -11) (-51.5, 0, -11) (-50.9142, 27.9142, -11) on bodies 3 in component "case rear"
ref_plane "WorkPlane1" through (-2.5, 0, 5.9) normal (1, 0, 0) x (0, 1, 0) in component "case front"
sketch "Sketch3 (3)" plane through (-2.5, 0, 5.6) normal (1, 0, 0) x (0, 1, 0) in component "case front"
  line L0 (27.5, -0.6) -> (27.5, -1.6)
  line L1 (-26.5, -0.6) -> (26.5, -0.6)
  line L2 (26.5971, -0.6) -> (25.0971, -0.6)
  line L3 (25.0971, -0.6) -> (25.5097, -3.8)
  line L4 (25.5097, -3.8) -> (26.5971, -3.8)
  line L5 (26.5971, -3.8) -> (26.5971, -0.6)
  line L6 (25.6, -3.0789) -> (26.7, -3.0789) construction
  line L7 (26.2971, -2.2066) -> (26.2971, -1.3) construction
  circle A0 centre (26.2971, -3.0789) radius 0.781
  line L8 (26.5, -0.6) -> (-26.5, -0.6)
  line L9 (0, -0.6) -> (0, 4.4) construction
  line L10 (-25.0971, -0.6) -> (-25.5097, -3.8)
  line L11 (-26.2971, -2.2066) -> (-26.1739, -0.589) construction
  line L12 (-25.5097, -3.8) -> (-26.5971, -3.8)
  line L13 (-26.5, -0.6) -> (-26.5, -1.6)
  line L14 (-26.5981, -0.6) -> (-25.0971, -0.6)
  line L15 (-25.6, -3.0789) -> (-26.7, -3.0789) construction
  circle A1 centre (-26.2971, -3.0789) radius 0.781
  line L16 (-26.5971, -3.8) -> (-26.5981, -0.6)
  line L17 (26.7, -0.6) -> (26.7, -1.6)
  point P0 (-26.5, -0.6)
  point P1 (-26.5, -0.6)
  dimension "d148" = 1.5
  dimension "d149" = 3.2
  dimension "d152" = 5
  constraint horizontal L2
  constraint horizontal L4
  constraint vertical L5
  constraint coincident L6 A0.centre
  constraint coincident L7 A0.centre
  constraint coincident L4.end A0
  constraint midpoint L8 L9.start
  constraint perpendicular L8 L9
  constraint coincident L3.end L4.start
  constraint symmetric L2.end L9 L10.start
  constraint symmetric L3.end L9 L10.end
  constraint symmetric L4.end L9 L12.end
  constraint symmetric L6.start L9 L15.start
  constraint symmetric L6.end L9 L15.end
  constraint symmetric L7.start L9 L11.start
  constraint symmetric A0 L9 A1
  constraint collinear L2 L8
  measures "d148" distance of L2.start L2.end
  measures "d149" distance of L2.start L4.end
  measures "d152" distance of L9.start L9.end
extrude "Extrude5''" add sketch "Sketch3 (3)" along normal mid plane 75 contours L1 L8 L10 L12 L14 A1 L16 | A1 L16 | L12 A1 L16 | L1 L2 L3 L4 L5 A0 L8 | L4 L5 A0 | L5 A0 bodies 2 in component "case front"
sketch "Sketch4 (2)" plane through (-2.5, 0, 5.6) normal (1, 0, 0) x (0, 1, 0) in component "case rear"
  line L0 (26.7, -1.6) -> (26.7, -14.8)
  line L1 (26.5971, -3.8) -> (25.5097, -3.8)
  line L2 (27.7, -1.6) -> (26.5, -1.6)
  line L3 (26.7, -1.6) -> (26.9, -1.6)
  line L4 (26.7, -1.6) -> (26.7, -2.15)
  line L5 (26.7, -2.15) -> (26.9, -1.6)
  line L6 (0, -0.6) -> (0, 4.4)
  line L7 (-26.7, -1.6) -> (-26.9, -1.6)
  line L8 (-26.7, -1.6) -> (-26.7, -2.15)
  line L9 (-26.7, -2.15) -> (-26.9, -1.6)
  line L10 (-26.7, -1.6) -> (-26.7, -14.8)
  circle A0 centre (26.2971, -3.0789) radius 0.781
  circle A1 centre (26.2971, -3.0789) radius 0.831
  circle A2 centre (-26.2971, -3.0789) radius 0.831
  line L11 (-26.7, -1.6) -> (-26.7, -14.8)
  point P0 (-26.5, -1.6)
  point P1 (26.5971, -2.3578)
  point P2 (26.5971, -0.6)
  dimension "d158" = 0.05
  constraint coincident L0.start L3.start
  constraint coincident L2 L3.end
  constraint perpendicular L0 L3
  constraint coincident L0 L4.end
  constraint symmetric L0.start L6 L7.start
  constraint symmetric L0.end L6 L10.end
  constraint symmetric L2.end L6 P0
  constraint symmetric L3.end L6 L7.end
  constraint symmetric L4.end L6 L8.end
  constraint symmetric L6 A1 A2
extrude "Extrude6'" cut sketch "Sketch4 (2)" along normal mid plane 76 contours L0 L2 L3 L4 L5 | L0 A0 A1 | L0 A0 | L7 L8 L9 L10 L11 | L10 A2 L11 picked at (-26.8255, -3.1751) bodies 3 in component "case rear"
fillet "Fillet1" radius 1.2 4 edges at (-42.3564, 19.6982, 5) (-42.3564, -22.3018, 5) (35.6436, -22.3018, 5) (35.6436, 19.6982, 5) on bodies 2 in component "case front"
sketch "Sketch5 (2)" plane through (0, -28.5, 0) normal (0, -1, 0) x (1, 0, 0) in component "case rear"
  line L0 (-49.5, -10.4) -> (44.5, -10.4)
  line L1 (44.5, -10.4) -> (44.5, 4.9)
  line L2 (44.5, 4.9) -> (-49.5, 4.9)
  line L3 (-49.5, 4.9) -> (-49.5, -10.4)
  line L4 (-2.6, 0) -> (-2.6, -1.8)
  line L5 (12.4, -1.8) -> (-2.6, -1.8)
  line L6 (12.4, 0) -> (-2.6, 0)
  line L7 (-2.6, 0) -> (-2.6, -1.8)
  line L8 (-2.6, -1.8) -> (12.4, -1.8)
  line L9 (12.4, -1.8) -> (12.4, 0)
  line L10 (-2.8, -3.4) -> (12.6, -3.4) construction
  line L11 (13.6, -2.4) -> (13.6, -0.2)
  line L12 (12.6, 0.8) -> (-2.8, 0.8)
  line L13 (-3.8, -0.2) -> (-3.8, -2.4)
  arc A0 (-2.8, 0.8) -> (-3.8, -0.2) centre (-2.8, -0.2) ccw
  arc A1 (13.6, -0.2) -> (12.6, 0.8) centre (12.6, -0.2) ccw
  arc A2 (12.6, -3.4) -> (13.6, -2.4) centre (12.6, -2.4) ccw
  arc A3 (-3.8, -2.4) -> (-2.8, -3.4) centre (-2.8, -2.4) ccw
  line L14 (0.9, -3.4) -> (8.9, -3.4)
  line L15 (8.9, -3.8) -> (8.9, -4.1)
  line L16 (8.4, -4.6) -> (1.4, -4.6)
  line L17 (0.9, -4.1) -> (0.9, -3.8)
  arc A4 (0.9, -4.1) -> (1.4, -4.6) centre (1.4, -4.1) ccw
  arc A5 (8.4, -4.6) -> (8.9, -4.1) centre (8.4, -4.1) ccw
  line L18 (12.6, -3.4) -> (9.3, -3.4)
  line L19 (0.5, -3.4) -> (-2.8, -3.4)
  arc A6 (9.3, -3.4) -> (8.9, -3.8) centre (9.3, -3.8) ccw
  arc A7 (0.9, -3.8) -> (0.5, -3.4) centre (0.5, -3.8) ccw
  point P0 (0.9, -4.6)
  point P1 (4.9, -3.4)
  dimension "d164" = 1
  dimension "d165" = 1
  dimension "d166" = 1
  dimension "d167" = 1
  dimension "d168" = 8
  dimension "d169" = 1.2
  dimension "d170" = 0.5
  dimension "d171" = 0.5
  dimension "d246" = 0.4
  dimension "d247" = 0.4
  constraint tangent L13 A0
  constraint tangent L12 A0
  constraint tangent L12 A1
  constraint tangent L11 A1
  constraint tangent L11 A2
  constraint tangent L10 A2
  constraint tangent L10 A3
  constraint tangent L13 A3
  constraint horizontal L14
  constraint vertical L15
  constraint horizontal L16
  constraint vertical L17
  constraint midpoint L14 P1
  constraint midpoint L10 P1
  constraint coincident P0 L17
  constraint coincident P0 L16
  constraint tangent L17 A4
  constraint tangent L16 A4
  constraint tangent L16 A5
  constraint tangent L15 A5
  constraint coincident L14.end L18
  constraint coincident L14.end L15
  constraint tangent L18 A6
  constraint tangent L15 A6
  constraint coincident L14.start L19
  constraint coincident L14.start L17
  constraint tangent L19 A7
  constraint tangent L17 A7
  measures "d164" radius of A0
  measures "d165" radius of A1
  measures "d166" radius of A2
  measures "d167" radius of A3
  measures "d168" distance of L14.start L14.end
  measures "d169" distance of L14.start P0
  measures "d170" radius of A4
  measures "d171" radius of A5
  measures "d246" radius of A6
  measures "d247" radius of A7
extrude "Extrude7'" cut sketch "Sketch5 (2)" against normal up to surface (1.8 mm away) contours L4 L5 L6 L7 L8 L9 | L11 L12 L13 A0 A1 A2 A3 L15 L16 L17 A4 A5 L18 L19 A6 A7 bodies 3 in component "case rear"
sketch "Sketch6 (2)" plane through (0, 0, -0.1) normal (0, 0, 1) x (-1, 0, 0) in component "case rear"
  circle A0 centre (-39, 21) radius 3.4
  circle A1 centre (-39, -21) radius 3.4
  circle A2 centre (44, 21) radius 3.4
  circle A3 centre (44, -21) radius 3.4
  line L0 (-39, -21) -> (44, -21) construction
  line L1 (44, -21) -> (44, 21) construction
  line L2 (44, 21) -> (-39, 21) construction
  line L3 (-39, 21) -> (-39, -21) construction
  line L4 (2.5, 21) -> (2.5, -21) construction
  line L5 (-39, 0) -> (44, 0) construction
  circle A4 centre (-39, 21) radius 1.7
  circle A5 centre (44, 21) radius 1.7
  circle A6 centre (44, -21) radius 1.7
  circle A7 centre (-39, -21) radius 1.7
  circle A8 centre (-39, 21) radius 2.3
  circle A9 centre (44, 21) radius 2.3
  circle A10 centre (-39, -21) radius 2.3
  circle A11 centre (44, -21) radius 2.3
  point P0 (-39, 21)
  dimension "d175" = 3.4
  dimension "d184" = 4.6
  constraint coincident P0 A0.centre
  constraint horizontal L0
  constraint vertical L1
  constraint horizontal L2
  constraint vertical L3
  constraint coincident A2.centre L1.end
  constraint coincident A1.centre L0.start
  constraint midpoint L2 L4.start
  constraint midpoint L0 L4.end
  constraint midpoint L3 L5.start
  constraint midpoint L1 L5.end
  constraint concentric A0 A4
  constraint symmetric L4 A4 A5
  constraint symmetric L5 A4 A7
  constraint symmetric L5 A5 A6
  constraint symmetric L4 A8 A9
  constraint symmetric L5 A8 A10
  constraint symmetric L5 A9 A11
  measures "d175" diameter of A4
  measures "d184" diameter of A8
extrude "Extrude8'" cut sketch "Sketch6 (2)" against normal up to surface (10.9 mm away) contours A4 | A5 | A6 | A7 bodies 3 in component "case rear"
extrude "Extrude9'" cut sketch "Sketch6 (2)" against normal blind 5 contours A4 | A5 | A6 | A8 | A9 | A10 | A11 bodies 3 in component "case rear"
extrude "Extrude12'" cut sketch "Sketch2 (3)" against normal up to surface (1.8 mm away) contours A12 L12 A20 | A12 A15 L12 L13 L14 L15 A20 A21 A22 A23 | A15 L14 A21 picked at (-38.5254, -20.5981) picked at (-38.5254, 20.5981) bodies 3 in component "case rear"
fillet "Fillet1'" radius 1.2 4 edges at (35.8301, 19.7705, -9.2) (35.8301, -22.2295, -9.2) (-47.1699, -22.2295, -9.2) (-47.1699, 19.7705, -9.2) on bodies 3 in component "case rear"
sketch "Sketch1 (4)" plane through (0, 0, -11) normal (0, 0, -1) x (1, 0, 0) in component "case back panel"
  line L0 (-49.5, -27.9) -> (44.5, -27.9)
  arc A0 (44.5, -27.9) -> (45.9, -26.5) centre (44.5, -26.5) ccw
  line L1 (45.9, -26.5) -> (45.9, 26.5)
  arc A1 (45.9, 26.5) -> (44.5, 27.9) centre (44.5, 26.5) ccw
  line L2 (44.5, 27.9) -> (-49.5, 27.9)
  arc A2 (-49.5, 27.9) -> (-50.9, 26.5) centre (-49.5, 26.5) ccw
  line L3 (-50.9, 26.5) -> (-50.9, -26.5)
  arc A3 (-50.9, -26.5) -> (-49.5, -27.9) centre (-49.5, -26.5) ccw
  line L4 (44.5, 26.7) -> (-49.5, 26.7)
  line L5 (-49.7, 26.5) -> (-49.7, -26.5)
  line L6 (-49.5, -26.7) -> (44.5, -26.7)
  line L7 (44.7, -26.5) -> (44.7, 26.5)
  arc A4 (44.5, -26.7) -> (44.7, -26.5) centre (44.5, -26.5) ccw
  arc A5 (-49.7, -26.5) -> (-49.5, -26.7) centre (-49.5, -26.5) ccw
  arc A6 (-49.5, 26.7) -> (-49.7, 26.5) centre (-49.5, 26.5) ccw
  arc A7 (44.7, 26.5) -> (44.5, 26.7) centre (44.5, 26.5) ccw
  line L8 (-48.5, 24.3) -> (-48.5, -24.3)
  line L9 (-47.3, -25.5) -> (42.3, -25.5)
  line L10 (43.5, -24.3) -> (43.5, 24.3)
  line L11 (42.3, 25.5) -> (-47.3, 25.5)
  arc A8 (43.5, 24.3) -> (42.3, 25.5) centre (42.3, 24.3) ccw
  arc A9 (-47.3, 25.5) -> (-48.5, 24.3) centre (-47.3, 24.3) ccw
  arc A10 (-48.5, -24.3) -> (-47.3, -25.5) centre (-47.3, -24.3) ccw
  arc A11 (42.3, -25.5) -> (43.5, -24.3) centre (42.3, -24.3) ccw
  arc A12 (-44, 16) -> (-39, 21) centre (-44, 21) ccw
  line L12 (-39, 21) -> (34, 21)
  arc A13 (34, 21) -> (39, 16) centre (39, 21) ccw
  line L13 (39, 16) -> (39, -16)
  arc A14 (39, -16) -> (34, -21) centre (39, -21) ccw
  line L14 (34, -21) -> (-39, -21)
  arc A15 (-39, -21) -> (-44, -16) centre (-44, -21) ccw
  line L15 (-44, -16) -> (-44, 16)
  line L16 (38.8, 15.8038) -> (38.8, -15.8038)
  arc A16 (38.8, -15.8038) -> (33.8038, -20.8) centre (39, -21) ccw
  line L17 (33.8038, -20.8) -> (-38.8038, -20.8)
  arc A17 (-38.8038, -20.8) -> (-43.8, -15.8038) centre (-44, -21) ccw
  line L18 (-43.8, -15.8038) -> (-43.8, 15.8038)
  arc A18 (-43.8, 15.8038) -> (-38.8038, 20.8) centre (-44, 21) ccw
  line L19 (-38.8038, 20.8) -> (33.8038, 20.8)
  arc A19 (33.8038, 20.8) -> (38.8, 15.8038) centre (39, 21) ccw
  line L20 (32.755, -19.6) -> (-37.755, -19.6)
  arc A20 (-37.755, -19.6) -> (-42.6, -14.755) centre (-44, -21) ccw
  line L21 (-42.6, -14.755) -> (-42.6, 14.755)
  arc A21 (-42.6, 14.755) -> (-37.755, 19.6) centre (-44, 21) ccw
  line L22 (-37.755, 19.6) -> (32.755, 19.6)
  arc A22 (32.755, 19.6) -> (37.6, 14.755) centre (39, 21) ccw
  line L23 (37.6, 14.755) -> (37.6, -14.755)
  arc A23 (37.6, -14.755) -> (32.755, -19.6) centre (39, -21) ccw
  circle A24 centre (39, 21) radius 1.7
  circle A25 centre (39, -21) radius 1.7
  circle A26 centre (-44, -21) radius 1.7
  circle A27 centre (-44, 21) radius 1.7
  line L24 (-34.4, -21.7) -> (-32.9, -21.7)
  line L25 (-32.9, -21.7) -> (-32.9, -18.7)
  line L26 (-32.9, -18.7) -> (-34.4, -18.7)
  line L27 (-34.4, -18.7) -> (-34.4, -21.7)
  line L28 (-28.9, -18.7) -> (-30.4, -18.7)
  line L29 (-30.4, -18.7) -> (-30.4, -21.7)
  line L30 (-30.4, -21.7) -> (-28.9, -21.7)
  line L31 (-28.9, -21.7) -> (-28.9, -18.7)
  line L32 (-34.4, -18.7) -> (-32.9, -18.7)
  line L33 (-32.9, -18.7) -> (-32.9, -21.7)
  line L34 (-32.9, -21.7) -> (-34.4, -21.7)
  line L35 (-34.4, -21.7) -> (-34.4, -18.7)
  line L36 (-30.4, -18.7) -> (-28.9, -18.7)
  line L37 (-28.9, -18.7) -> (-28.9, -21.7)
  line L38 (-28.9, -21.7) -> (-30.4, -21.7)
  line L39 (-30.4, -21.7) -> (-30.4, -18.7)
  dimension "d206" = 1.2
  dimension "d207" = 1.2
  dimension "d208" = 1.2
  dimension "d209" = 1.2
  dimension "d229" = 0.2
  dimension "d230" = 1.4
  constraint tangent L11 A8
  constraint tangent L10 A8
  constraint tangent L8 A9
  constraint tangent L11 A9
  constraint tangent L8 A10
  constraint tangent L9 A10
  constraint tangent L9 A11
  constraint tangent L10 A11
  constraint horizontal L32
  constraint vertical L33
  constraint horizontal L34
  constraint vertical L35
  constraint coincident L24.end L25.start
  constraint coincident L26.end L27.start
  constraint horizontal L36
  constraint vertical L37
  constraint horizontal L38
  constraint vertical L39
  constraint coincident L30.end L31.start
  constraint coincident L28.end L29.start
  measures "d206" radius of A8
  measures "d207" radius of A9
  measures "d208" radius of A10
  measures "d209" radius of A11
extrude "Extrude1'''" add sketch "Sketch1 (4)" along normal blind 1.8 separate body contours L8 L9 L10 L11 A8 A9 A10 A11 | A12 L12 A13 L13 A14 L14 A15 L15 L16 A16 L17 A17 L18 A18 L19 A19 L27 L31 L35 L37 | L14 L17 L25 L27 L33 L35 | L14 L24 L25 L27 L33 L34 L35 | L14 L17 L25 L29 L33 L39 | L17 L20 L25 L27 L33 L35 | L16 A16 L17 A17 L18 A18 L19 A19 L20 A20 L21 A21 L22 A22 L23 A23 L27 L31 L35 L37 | L14 L17 L29 L31 L37 L39 | L14 L29 L30 L31 L37 L38 L39 | L17 L20 L25 L29 L33 L39 | L20 L25 L26 L27 L32 L33 L35 | L20 A20 L21 A21 L22 A22 L23 A23 L25 L26 L27 L28 L29 L31 L32 L33 L35 L36 L37 L39 | L17 L20 L29 L31 L37 L39 | L20 L28 L29 L31 L36 L37 L39 | A24 | A25 | A26 | A27 makes body 8 in component "case back panel"
extrude "Extrude3'''" cut sketch "Sketch1 (4)" along normal up to surface (1.4 mm away) contours A24 | A25 | A26 | A27 bodies 8 in component "case back panel"
extrude "Extrude2'''" add sketch "Sketch1 (4)" against normal blind 0.4 contours L17 L20 L25 L27 L33 L35 | L16 A16 L17 A17 L18 A18 L19 A19 L20 A20 L21 A21 L22 A22 L23 A23 L27 L31 L35 L37 | L17 L20 L25 L29 L33 L39 | L17 L20 L29 L31 L37 L39 bodies 8 in component "case back panel"
extrude "Extrude4'''" cut sketch "Sketch1 (4)" along normal up to surface (1.8 mm away) contours L20 L25 L26 L27 L32 L33 L35 | L20 L28 L29 L31 L36 L37 L39 bodies 8 in component "case back panel"
fillet "Fillet1''" radius 0.4 16 edges at (33.8038, 20.8, -10.8) (-43.8, -15.8038, -10.8) (-43.8, 15.8038, -10.8) (-42.6, 14.755, -10.8) (37.6, -14.755, -10.8) (33.8038, -20.8, -10.8) (-37.755, -19.6, -10.8) (-37.755, 19.6, -10.8) (32.755, 19.6, -10.8) (38.8, 15.8038, -10.8) (37.6, 14.755, -10.8) (-42.6, -14.755, -10.8) (38.8, -15.8038, -10.8) (32.755, -19.6, -10.8) (-38.8038, -20.8, -10.8) (-38.8038, 20.8, -10.8) on bodies 8 in component "case back panel"
chamfer "Chamfer1''" distance 0.6 angle 45 8 edges at (-48.5, 0, -12.8) (-48.1485, 25.1485, -12.8) (-2.5, 25.5, -12.8) (43.1485, 25.1485, -12.8) (43.5, 0, -12.8) (43.1485, -25.1485, -12.8) (-2.5, -25.5, -12.8) (-48.1485, -25.1485, -12.8) on bodies 8 in component "case back panel"
sketch "Sketch1 (5)" plane through (46.5, 0, 0) normal (1, 0, 0) x (0, 1, 0) in component "case foot"
  line L0 (-26.5, -10.4) -> (26.5, -10.4)
  line L1 (26.5, -10.4) -> (26.5, 4.9)
  line L2 (26.5, 4.9) -> (-26.5, 4.9)
  line L3 (-26.5, 4.9) -> (-26.5, -10.4)
  line L4 (-14.1, 2.5) -> (-4.5, 2.5)
  arc A0 (-2.9, 0.9) -> (-4.5, 2.5) centre (-4.5, 0.9) ccw
  line L5 (-2.9, 0.9) -> (-2.9, -3.4)
  arc A1 (-4.5, -5) -> (-2.9, -3.4) centre (-4.5, -3.4) ccw
  line L6 (-4.5, -5) -> (-14.1, -5)
  arc A2 (-15.7, -3.4) -> (-14.1, -5) centre (-14.1, -3.4) ccw
  line L7 (-15.7, -3.4) -> (-15.7, 0.9)
  arc A3 (-14.1, 2.5) -> (-15.7, 0.9) centre (-14.1, 0.9) ccw
  line L8 (-26.5, -11) -> (26.5, -11)
  line L9 (28.5, 4.9) -> (28.5, -10.4)
  line L10 (22.7, -5.1) -> (19.3, -5.1)
  line L11 (-26.5, -11) -> (28.5, -11) construction
  line L12 (28.5, -11) -> (28.5, 4.9) construction
  line L13 (28.5, 4.9) -> (-26.5, 4.9) construction
  line L14 (-26.5, 4.9) -> (-26.5, -11) construction
  line L15 (21, -5.1) -> (21, -11) construction
  line L16 (17, -12.8) -> (28.7, -12.8)
  line L17 (28.7, -12.8) -> (28.7, -19.8)
  line L18 (28.7, -19.8) -> (17, -19.8)
  line L19 (17, -19.8) -> (17, -12.8)
  line L20 (25.6, -12.8) -> (28.7, -12.8)
  line L21 (28.7, -12.8) -> (28.7, -11.2)
  line L22 (28.7, -11.2) -> (25.6, -11.2)
  line L23 (25.6, -11.2) -> (25.6, -12.8)
  line L24 (25.5, -11) -> (25.5, -12.2)
  line L25 (-24.3, -12.8) -> (24.3, -12.8)
  line L26 (28.7, -19.8) -> (34.7, -19.8)
  line L27 (34.7, -19.8) -> (34.7, 4.9)
  line L28 (34.7, 4.9) -> (28.7, 4.9)
  line L29 (28.7, 4.9) -> (28.7, -19.8)
  line L30 (28.7, 4.9) -> (68.7, 4.9)
  line L31 (68.7, 4.9) -> (68.7, -1.1)
  line L32 (68.7, -1.1) -> (28.7, -1.1)
  line L33 (28.7, -1.1) -> (28.7, 4.9)
  line L34 (69.9941, 9.7296) -> (73.8578, 8.6944)
  line L35 (73.8578, 8.6944) -> (60.9168, -39.6019)
  line L36 (60.9168, -39.6019) -> (57.0531, -38.5667)
  line L37 (57.0531, -38.5667) -> (69.9941, 9.7296)
  dimension "d187" = 7
  dimension "d188" = 4
  dimension "d218" = 1.8
  dimension "d225" = 1.6
  dimension "d226" = 0.1
  dimension "d239" = 0.2
  dimension "d240" = 6
  dimension "d244" = 4
  dimension "d245" = 50
  dimension "d248" = 40
  constraint horizontal L11
  constraint vertical L12
  constraint horizontal L13
  constraint vertical L14
  constraint coincident L9.start L12.end
  constraint coincident L8.start L11.start
  constraint midpoint L10 L15.start
  constraint perpendicular L11 L15
  constraint horizontal L16
  constraint vertical L17
  constraint horizontal L18
  constraint vertical L19
  constraint horizontal L20
  constraint vertical L21
  constraint horizontal L22
  constraint vertical L23
  constraint coincident L16 L20.start
  constraint collinear L16 L25
  constraint coincident L16.end L17.start
  constraint collinear L17 L21
  constraint horizontal L26
  constraint vertical L27
  constraint horizontal L28
  constraint vertical L29
  constraint collinear L13 L28
  constraint perpendicular L30 L33
  constraint perpendicular L31 L32
  constraint perpendicular L34 L35
  constraint perpendicular L36 L37
  constraint coincident L29 L32.end
  measures "d187" distance of L16.start L18.end
  measures "d188" distance of L15 L19
  measures "d218" distance of L15.end L16
  measures "d225" distance of L20.start L22.end
  measures "d226" distance of L23 L24
  measures "d239" distance of L12 L21.end
  measures "d240" distance of L17.end L26.end
  measures "d244" distance of L34.start L34.end
  measures "d245" distance of L34.start L36.end
  measures "d248" distance of L31 L33
extrude "Extrude1''''" add sketch "Sketch1 (5)" along normal mid plane 10 separate body contours L16 L17 L18 L19 L20 L25 L29 | L16 L20 L21 L22 L23 L29 | L17 L21 L26 L27 L29 L32 | L27 L28 L29 L30 L32 L33 | L27 L30 L32 L37 | L31 L32 L37 | L31 L32 L34 L35 L36 L37 makes body 9 in component "case foot"
move_body "Move4" bodies 9 to x (1, 0, 0) y (0, 1, 0) z (0, 0, 1) at (-7.5, 0, 0) in component "case foot"
sketch "Sketch3 (4)" plane through (0, 0, -19.8) normal (0, 0, -1) x (1, 0, 0) in component "case foot"
  line L0 (44, -34.7) -> (44, -17)
  line L1 (44, -17) -> (34, -17)
  line L2 (34, -17) -> (34, -34.7)
  circle A0 centre (39, -21) radius 3
  circle A1 centre (39, -21) radius 1.7
  line L3 (34, -34.7) -> (44, -34.7)
  dimension "d219" = 6
  measures "d219" diameter of A0
extrude "Extrude4''''" cut sketch "Sketch3 (4)" against normal up to surface (7 mm away) contours A1 bodies 9 in component "case foot"
extrude "Extrude5'''" cut sketch "Sketch3 (4)" against normal blind 3 contours A0 | A1 bodies 9 in component "case foot"
chamfer "Chamfer3" distance 0.4 angle 45 33 edges at (34, 25.6, -12) (34, 34.7, -10.45) (44, 25.6, -12) (34, 67.3873, -15.4538) (44, 34.7, -10.45) (44, 67.3873, -15.4538) (34, 62.0727, -19.8333) (44, 62.0727, -19.8333) (34, 48.7, 4.9) (34, 25.85, -19.8) (44, 48.7, 4.9) (44, 71.9259, 9.212) (34, 71.9259, 9.212) (39, 28.7, 4.9) (39, 73.8578, 8.6944) (44, 21.3, -12.8) (34, 50.8962, -1.1) (44, 27.15, -11.2) (34, 28.7, -3.15) (39, 60.9168, -39.6019) (34, 27.15, -11.2) (44, 28.7, -3.15) (44, 50.8962, -1.1) (44, 25.85, -19.8) (34, 21.3, -12.8) (44, 58.985, -39.0843) (39, 34.7, -19.8) (39, 17, -19.8) (39, 17, -12.8) (44, 17, -16.3) (34, 58.985, -39.0843) (39, 57.0531, -38.5667) (34, 17, -16.3) on bodies 9 in component "case foot"
component "Display" placed x (1, 0, 0) y (0, 1, 0) z (0, 0, 1) at (0, 0, 0)
component "case front" placed x (1, 0, 0) y (0, 1, 0) z (0, 0, 1) at (0, 0, 0)
component "case rear" placed x (1, 0, 0) y (0, 1, 0) z (0, 0, 1) at (0, 0, 0)